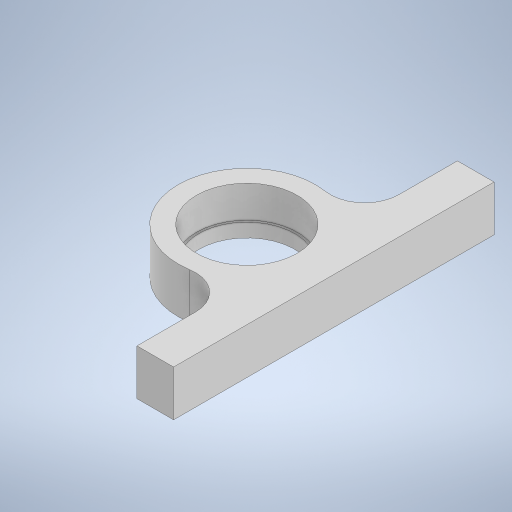
# Autodesk Inventor part: Bearing Holder
Saved by Autodesk Inventor 2023 (Build 270158000, 158)
## iProperties
Created: 2022-10-18
Part Number: Bearing Holder
Material: Generic
Document SubType Name: Modeling
Designer: neera
Density: 1 g/cm^3
Appearance: Default
Author: neera
Autodesk Inventor part; units mm, degrees
ref_plane "YZ Plane" through (0, 0, 0) normal (1, 0, 0) x (0, 1, 0)
ref_plane "XZ Plane" through (0, 0, 0) normal (0, 1, 0) x (-1, 0, 0)
ref_plane "XY Plane" through (0, 0, 0) normal (0, 0, 1) x (1, 0, 0)
sketch "Sketch1" plane through (0, 0, 0) normal (0, 1, 0) x (-1, 0, 0)
  line L0 (4, 35) -> (-4, 35)
  line L1 (-4, 35) -> (-4, -35)
  line L2 (-4, -35) -> (4, -35)
  line L3 (4, -35) -> (4, 35)
  line L4 (4, 35) -> (-4, -35) construction
  line L5 (-4, 35) -> (4, -35) construction
  circle A0 centre (15, 0) radius 15
  arc A1 (4, 22.2261) -> (12.6667, 14.8174) centre (11.5, 22.2261) ccw
  arc A2 (12.6667, -14.8174) -> (4, -22.2261) centre (11.5, -22.2261) ccw
  point P0 (0, 0)
  dimension "d0" = 8
  dimension "d1" = 70
  dimension "d2" = 30
  dimension "d3" = 15
  dimension "d6" = 15
  dimension "d7" = 7.5
  dimension "d9" = 0
  dimension "d10" = 15
  constraints: 12 end point, 6 point on circle, 3 centre point, 3 tangent, 2 midpoint, 2 parallel, 2 point on line, 1 horizontal, 1 perpendicular
  measures "d0" distance of L2.end L1.end
  measures "d1" distance of L1.end L0.end
  measures "d2" diameter of A0
  measures "d3" distance of A0.centre point (0, 0)
  measures "d6" diameter of A1
  measures "d7" distance from line of L3 A1.centre
  measures "d9" vertical distance of A0.centre point (0, 0)
  measures "d10" diameter of A2
extrude "Extrusion1" add sketch "Sketch1" along normal blind 10
sketch "Sketch2" plane through (0, 10, 0) normal (0, 1, 0) x (1, 0, 0)
  circle A0 centre (-15, 0) radius 11
  arc A1 (-12.6667, 14.8174) -> (-12.6667, -14.8174) centre (-15, 0) ccw projected
  point P0 (0, 0)
  dimension "d13" = 22
  constraints: 1 centre point, 1 concentric
  measures "d13" diameter of A0
extrude "Extrusion2" cut sketch "Sketch2" against normal blind 7
sketch "Sketch3" plane through (-15, 3, 0) normal (0, 1, 0) x (1, 0, 0)
  circle A0 centre (0, 0) radius 10.5
  point P0 (15, 0)
  dimension "d16" = 21
  constraints: 1 centre point
  measures "d16" diameter of A0
extrude "Extrusion3" cut sketch "Sketch3" against normal blind 7
sketch "Sketch4" plane through (-4, 0, 22.2261) normal (-1, 0, 0) x (0, 0, 1)
  circle A0 centre (6.7739, 5) radius 3
  line L0 (0, 0) -> (12.7739, 0) projected
  line L1 (12.7739, 0) -> (12.7739, 10) projected
  circle A1 centre (-51.2261, 5) radius 3
  line L2 (-57.2261, 10) -> (-44.4522, 10) projected
  line L3 (-57.2261, 0) -> (-57.2261, 10) projected
  point P0 (-22.2261, 0)
  point P1 (6.3869, 0)
  dimension "d19" = 6
  dimension "d20" = 5
  dimension "d21" = 6
  dimension "d22" = 6
  dimension "d23" = 5
  dimension "d24" = 6
  constraints: 2 centre point, 1 midpoint
  measures "d19" diameter of A0
  measures "d20" vertical distance of point (6.387, 0) A0.centre
  measures "d21" distance from line of L1 A0.centre
  measures "d22" diameter of A1
  measures "d23" distance from line of L2 A1.centre
  measures "d24" distance from line of L3 A1.centre
extrude "Extrusion4" cut sketch "Sketch4" against normal blind 7
body "Solid1"
